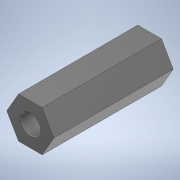
# Autodesk Inventor part: MainboardSpacer
Saved by Autodesk Inventor 2020 (Build 240168000, 168)
## iProperties
Created: 2019-08-14
Part Number: MainboardSpacer
Material: Generic
Document SubType Name: Modeling
Designer: victo
Density: 1 g/cm^3
Appearance: Default
Author: victo
Autodesk Inventor part; units mm, degrees
ref_plane "YZ Plane" through (0, 0, 0) normal (1, 0, 0) x (0, 1, 0)
ref_plane "XZ Plane" through (0, 0, 0) normal (0, 1, 0) x (-1, 0, 0)
ref_plane "XY Plane" through (0, 0, 0) normal (0, 0, 1) x (1, 0, 0)
sketch "Sketch1" plane through (0, 0, 0) normal (0, 0, 1) x (1, 0, 0)
  circle A0 centre (0, 0) radius 1.5
  line L0 (-1.7321, -3) -> (-3.4641, 0)
  line L1 (-3.4641, 0) -> (-1.7321, 3)
  line L2 (-1.7321, 3) -> (1.7321, 3)
  line L3 (1.7321, 3) -> (3.4641, 0)
  line L4 (3.4641, 0) -> (1.7321, -3)
  line L5 (1.7321, -3) -> (-1.7321, -3)
  dimension "d0" = 3
  dimension "d1" = 3
  constraints: 12 end point, 2 coincident, 1 centre point, 1 horizontal, 13 other
  measures "d0" diameter of A0
  measures "d1" distance from line of L5 point (0, 0)
extrude "Extrusion1" add sketch "Sketch1" along normal blind 17.5
body "Solid1"
